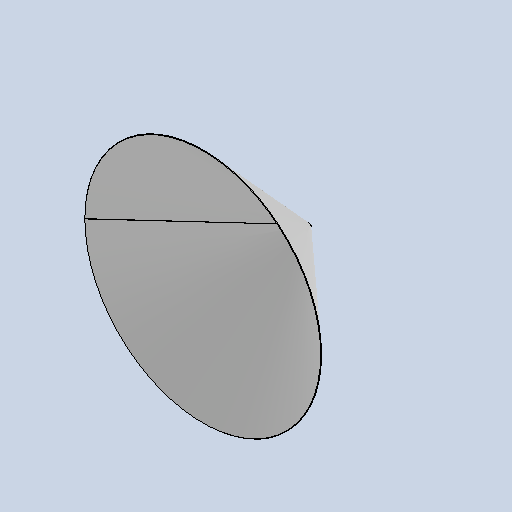
# Autodesk Inventor part: MSC 103 roсket nose
Saved by Autodesk Inventor 2025 (Build 290162010, 162A)
## iProperties
Created: 2024-05-19
Part Number: MSC 103 roсket nose
Material: Stainless Steel
Document SubType Name: Sheet Metal
Designer: admin
Density: 8 g/cm^3
Flat Pattern Width: 40.4568 cm
Flat Pattern Length: 40.5057 cm
Flat Pattern Area: 1638.73 cm^2
Sheet Metal Rule: Default
Sheet Metal Width: 404,568 mm
Sheet Metal Length: 405,057 mm
Sheet Metal Area: 163873,073 mm^2
Appearance: Default
Stock Number: МОО 103 ракета нос
Author: admin
Autodesk Inventor part; units mm, degrees
ref_plane "YZ Plane" through (0, 0, 0) normal (1, 0, 0) x (0, 1, 0)
ref_plane "XZ Plane" through (0, 0, 0) normal (0, 1, 0) x (-1, 0, 0)
ref_plane "XY Plane" through (0, 0, 0) normal (0, 0, 1) x (1, 0, 0)
sketch "Sketch1" plane through (0, 0, 0) normal (0, 0, 1) x (1, 0, 0)
  line L0 (-149.4612, 0) -> (-1.9612, 134.4087)
  line L1 (-1.9612, 134.4087) -> (-2.5, 135)
  line L2 (-2.5, 135) -> (-150, 0.5913)
  line L3 (-150, 0.5913) -> (-149.4612, 0)
  line L4 (-149.4612, 0) -> (-2.5, 135) construction
  line L5 (-1.9612, 134.4087) -> (-150, 0.5913) construction
  line L6 (0, 0) -> (0, 135)
  point P0 (-75.9806, 67.5)
  dimension "d0" = 0.8
  dimension "d3" = 300
  dimension "d4" = 135
  dimension "d5" = 5
  constraints: 14 end point, 2 horizontal alignment, 2 midpoint, 2 parallel, 1 perpendicular, 1 vertical
  measures "d0" distance of L0.end L1.end
  measures "d3" diameter of L2.end L6
  measures "d4" distance of L6.start L6.end
  measures "d5" diameter of L1.end L6
revolve "Revolution1" add sketch "Sketch1" angle 359.9 about axis through (0, 0, 0) along (0, 1, 0)
equation "\"d0\" = Thickness"
equation "\"BendRadius\" = Thickness"
equation "\"BendReliefWidth\" = Thickness"
equation "\"BendReliefDepth\" = 0.5 * Thickness"
equation "\"CornerReliefSize\" = 4 * Thickness"
equation "\"MinimumRemnant\" = 2 * Thickness"
equation "\"TransitionRadius\" = BendRadius"
equation "\"JacobiRadiusSize\" = BendRadius"
equation "\"GapSize\" = Thickness"
equation "\"Thickness\" = 0.8"
body "Solid1"
